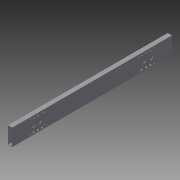
# Autodesk Inventor part: boxbeam 4x1 with sideways holes
Saved by Autodesk Inventor 2015 (Build 190159000, 159)
## iProperties
Created: 2015-01-31
Part Number: boxbeam 4x1 with sideways holes
Material: Generic
Document SubType Name: Modeling
Designer: szymsea16
Density: 1 g/cm^3
Appearance: Default
Author: szymsea16
Autodesk Inventor part; units mm, degrees
ref_plane "YZ Plane" through (0, 0, 0) normal (1, 0, 0) x (0, 1, 0)
ref_plane "XZ Plane" through (0, 0, 0) normal (0, 1, 0) x (-1, 0, 0)
ref_plane "XY Plane" through (0, 0, 0) normal (0, 0, 1) x (1, 0, 0)
sketch "Sketch1" plane through (0, 0, 0) normal (0, 1, 0) x (-1, 0, 0)
  line L0 (0, 0) -> (0, -965.2)
  line L1 (0, -965.2) -> (25.4, -965.2)
  line L2 (0, 0) -> (25.4, 0)
  line L3 (25.4, 0) -> (25.4, -965.2)
  dimension "d0" = 965.2
  dimension "d1" = 25.4
  dimension "d2" = 25.4
  dimension "d3" = 965.2
  constraints: 8 end point, 1 parallel, 1 perpendicular, 1 vertical
  measures "d0" distance of L0.start L0.end
  measures "d1" distance of L0.end L1.end
  measures "d2" distance of L0.start L2.end
  measures "d3" distance of L2.end L1.end
extrude "Extrusion1" add sketch "Sketch1" along normal blind 101.6
sketch "Sketch2" plane through (0, 0, -965.2) normal (0, 0, -1) x (-1, 0, 0)
  line L0 (0, 101.6) -> (25.4, 101.6) projected
  line L1 (22.225, 98.425) -> (3.175, 98.425)
  line L2 (3.175, 98.425) -> (3.175, 3.175)
  line L3 (3.175, 3.175) -> (22.225, 3.175)
  line L4 (22.225, 3.175) -> (22.225, 98.425)
  point P0 (0, 0)
  dimension "d8" = 19.05
  dimension "d9" = 95.25
  dimension "d10" = 19.05
  constraints: 8 end point, 2 perpendicular
  measures "d8" distance of L1.start L1.end
  measures "d9" distance of L1.end L2.end
  measures "d10" distance of L2.end L3.end
extrude "Extrusion2" cut sketch "Sketch2" against normal blind 2540
sketch "Sketch3" plane through (-25.4, 0, -965.2) normal (-1, 0, 0) x (0, 0, 1)
  line L0 (89.1033, 114.2993) -> (200.7415, 105.2475)
  arc A0 (206.5783, 98.9183) -> (200.7415, 105.2475) centre (200.2283, 98.9183) ccw
  line L1 (206.5783, 98.9183) -> (206.5783, 2.6802)
  arc A1 (200.7415, -3.649) -> (206.5783, 2.6802) centre (200.2283, 2.6802) ccw
  line L2 (200.7415, -3.649) -> (89.1033, -12.7007)
  line L3 (89.1033, -12.7007) -> (87.4523, -12.7007)
  line L4 (87.4523, 114.2993) -> (87.4523, -12.7007)
  line L5 (87.4523, 114.2993) -> (89.1033, 114.2993)
  circle A2 centre (108.688, 6.2223) radius 2.0447
  circle A3 centre (197.588, 88.3913) radius 2.0447
  circle A4 centre (108.688, 12.0643) radius 2.5527
  circle A5 centre (197.588, 82.5493) radius 2.5527
  circle A6 centre (180.57, 12.0643) radius 5.5562
  circle A7 centre (129.77, 12.0643) radius 5.5562
  circle A8 centre (180.57, 89.5343) radius 5.5562
  circle A9 centre (167.7163, 50.7993) radius 11.1061
  circle A10 centre (155.17, 89.5343) radius 5.5562
  circle A11 centre (129.77, 89.5343) radius 5.5562
  circle A12 centre (155.17, 12.0643) radius 5.5562
  circle A13 centre (127.0001, 50.7993) radius 14.2811
  circle A14 centre (197.588, 19.0493) radius 2.5527
  circle A15 centre (108.688, 89.5343) radius 2.5527
  circle A16 centre (197.588, 13.2073) radius 2.0447
  circle A17 centre (108.688, 95.3763) radius 2.0447
  circle A18 centre (197.588, 13.2073) radius 2.0447
  circle A19 centre (197.588, 19.0493) radius 2.5527
  circle A20 centre (197.588, 82.5493) radius 2.5527
  circle A21 centre (197.588, 88.3913) radius 2.0447
  circle A22 centre (167.7163, 50.7993) radius 11.1061
  circle A23 centre (180.57, 89.5343) radius 5.5563
  circle A24 centre (155.17, 89.5343) radius 5.5562
  circle A25 centre (129.77, 89.5343) radius 5.5562
  circle A26 centre (127.0001, 50.7993) radius 14.2811
  circle A27 centre (129.77, 12.0643) radius 5.5562
  circle A28 centre (155.17, 12.0643) radius 5.5562
  circle A29 centre (180.57, 12.0643) radius 5.5562
  circle A30 centre (108.688, 89.5343) radius 2.5527
  circle A31 centre (108.688, 95.3763) radius 2.0447
  circle A32 centre (108.688, 12.0643) radius 2.5527
  circle A33 centre (108.688, 6.2223) radius 2.0447
  line L6 (0, 101.6) -> (0, 50.8)
  line L7 (965.2, 101.6) -> (965.2, 50.8)
  line L8 (965.2, 3.175) -> (965.2, 98.425) projected
  line L9 (0, 50.8) -> (127, 50.8)
  line L10 (965.2, 50.8) -> (838.2, 50.8)
  line L11 (965.2, 101.6) -> (0, 101.6) projected
  line L12 (482.6, 101.6) -> (482.6, 3.175)
  circle A34 centre (767.612, 88.3913) radius 2.0447
  arc A35 (764.4585, 105.2475) -> (758.6217, 98.9183) centre (764.9717, 98.9183) ccw
  circle A36 centre (767.612, 82.5493) radius 2.5527
  circle A37 centre (767.612, 82.5493) radius 2.5527
  line L13 (758.6217, 98.9183) -> (758.6217, 2.6802)
  arc A38 (758.6217, 2.6802) -> (764.4585, -3.649) centre (764.9717, 2.6802) ccw
  circle A39 centre (767.612, 88.3913) radius 2.0447
  circle A40 centre (784.63, 89.5343) radius 5.5562
  circle A41 centre (784.63, 89.5343) radius 5.5563
  circle A42 centre (810.03, 89.5343) radius 5.5562
  circle A43 centre (810.03, 89.5343) radius 5.5562
  line L14 (764.4585, -3.649) -> (876.0967, -12.7007)
  line L15 (877.7477, 114.2993) -> (877.7477, -12.7007)
  circle A44 centre (835.43, 89.5343) radius 5.5562
  circle A45 centre (835.43, 89.5343) radius 5.5562
  line L16 (876.0967, 114.2993) -> (764.4585, 105.2475)
  circle A46 centre (856.512, 95.3763) radius 2.0447
  circle A47 centre (856.512, 95.3763) radius 2.0447
  circle A48 centre (856.512, 89.5343) radius 2.5527
  circle A49 centre (856.512, 89.5343) radius 2.5527
  line L17 (877.7477, 114.2993) -> (876.0967, 114.2993)
  line L18 (876.0967, -12.7007) -> (877.7477, -12.7007)
  circle A50 centre (856.512, 6.2223) radius 2.0447
  circle A51 centre (856.512, 12.0643) radius 2.5527
  circle A52 centre (856.512, 6.2223) radius 2.0447
  circle A53 centre (856.512, 12.0643) radius 2.5527
  circle A54 centre (835.43, 12.0643) radius 5.5562
  circle A55 centre (835.43, 12.0643) radius 5.5562
  circle A56 centre (838.1999, 50.7993) radius 14.2811
  circle A57 centre (838.1999, 50.7993) radius 14.2811
  circle A58 centre (810.03, 12.0643) radius 5.5562
  circle A59 centre (810.03, 12.0643) radius 5.5562
  circle A60 centre (784.63, 12.0643) radius 5.5562
  circle A61 centre (784.63, 12.0643) radius 5.5562
  circle A62 centre (767.612, 13.2073) radius 2.0447
  circle A63 centre (767.612, 13.2073) radius 2.0447
  circle A64 centre (767.612, 19.0493) radius 2.5527
  circle A65 centre (767.612, 19.0493) radius 2.5527
  circle A66 centre (797.4837, 50.7993) radius 11.1061
  circle A67 centre (797.4837, 50.7993) radius 11.1061
  point P0 (965.2, 0)
  point P1 (758.7399, 264.0927)
  point P2 (0, 76.2)
  dimension "d13" = 50.8
  dimension "d15" = 50.8
  dimension "d216" = 127
  dimension "d217" = 127
  constraints: 68 centre point, 42 symmetric about line, 34 end point, 12 equal radius, 8 point on circle, 4 parallel, 4 tangent, 3 horizontal, 3 midpoint, 1 vertical, 35 other
  measures "d13" distance of L6.start L6.end
  measures "d15" distance of L7.start L7.end
  measures "d216" distance of L6.end L9.end
  measures "d217" distance of L7.end L10.end
extrude "Extrusion7" cut sketch "Sketch3" against normal blind 2540 contours A13
extrude "Extrusion8" cut sketch "Sketch3" against normal blind 2540 contours A2 | A3 | A4 | A5 | A6 | A7 | A8 | A9 | A10 | A11 | A12 | A14 | A15 | A16 | A17
extrude "Extrusion11" cut sketch "Sketch3" against normal through all contours A56 | A13 | A2 | A3 | A4 | A5 | A6 | A7 | A8 | A9 | A10 | A11 | A12 | A14 | A15 | A16 | A17 | A34 | A36 | A40 | A42 | A44 | A46 | A48 | A50 | A51 | A54 | A58 | A60 | A62 | A64 | A66
body "Solid1"
